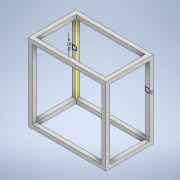
# Autodesk Inventor part: Battery housing
Saved by Autodesk Inventor 2020 (Build 240168000, 168)
## iProperties
Created: 2020-10-20
Part Number: Battery housing
Material: Generic
Document SubType Name: Modeling
Designer: jtri402
Density: 1 g/cm^3
Appearance: Default
Author: jtri402
Autodesk Inventor part; units mm, degrees
ref_plane "YZ Plane" through (0, 0, 0) normal (1, 0, 0) x (0, 1, 0)
ref_plane "XZ Plane" through (0, 0, 0) normal (0, 1, 0) x (-1, 0, 0)
ref_plane "XY Plane" through (0, 0, 0) normal (0, 0, 1) x (1, 0, 0)
sketch "Sketch1" plane through (0, 0, 0) normal (0, 0, 1) x (1, 0, 0)
  line L0 (0, 0) -> (175, 0)
  line L1 (175, 0) -> (175, 175)
  line L2 (175, 175) -> (0, 175)
  line L3 (0, 175) -> (0, 0)
  dimension "d0" = 175
  dimension "d1" = 175
  constraints: 8 end point, 2 parallel, 1 horizontal, 1 perpendicular
  measures "d0" distance of L2.end L0.start
  measures "d1" distance of L0.start L0.end
extrude "Extrusion1" add sketch "Sketch1" along normal blind 100
sketch "Sketch2" plane through (0, 175, 0) normal (0, 1, 0) x (1, 0, 0)
  line L0 (0, 0) -> (175, 0) projected
  line L1 (0, -100) -> (175, -100) projected
  line L2 (0, 0) -> (175, 0)
  line L3 (175, 0) -> (175, -100)
  line L4 (175, -100) -> (0, -100)
  line L5 (0, -100) -> (0, 0)
  line L6 (10, -10) -> (165, -10)
  line L7 (165, -10) -> (165, -90)
  line L8 (165, -90) -> (10, -90)
  line L9 (10, -90) -> (10, -10)
  dimension "d4" = 10
  dimension "d5" = 10
  dimension "d6" = 10
  dimension "d7" = 10
  constraints: 16 end point, 4 parallel, 2 horizontal, 2 perpendicular
  measures "d4" distance between parallel lines of L0 L6
  measures "d5" distance between parallel lines of L5 L9
  measures "d6" distance between parallel lines of L1 L8
  measures "d7" distance between parallel lines of L3 L7
extrude "Extrusion2" add sketch "Sketch2" along normal blind 10
sketch "Sketch3" plane through (10, 175, 10) normal (0, 1, 0) x (1, 0, 0)
  line L0 (0, -80) -> (0, 0) projected
  line L1 (0, -80) -> (155, -80) projected
  line L2 (0, 0) -> (155, 0)
  line L3 (155, 0) -> (155, -80)
  line L4 (155, -80) -> (0, -80)
  line L5 (0, -80) -> (0, 0)
  point P0 (-10, 10)
  constraints: 8 end point, 2 parallel, 1 horizontal, 1 perpendicular
extrude "Extrusion3" cut sketch "Sketch3" against normal blind 9000
sketch "Sketch4" plane through (0, 0, 100) normal (0, 0, 1) x (1, 0, 0)
  line L0 (175, 0) -> (175, 185) projected
  line L1 (175, 185) -> (195, 185)
  line L2 (195, 185) -> (195, 0)
  line L3 (195, 0) -> (175, 0)
  line L4 (175, 0) -> (175, 185)
  point P0 (0, 0)
  dimension "d12" = 20
  constraints: 8 end point, 2 parallel, 1 horizontal, 1 perpendicular
  measures "d12" distance of L2.end L3.end
extrude "Extrusion4" add sketch "Sketch4" against normal blind 100
sketch "Sketch5" plane through (0, 0, 100) normal (0, 0, 1) x (1, 0, 0)
  line L0 (10, 175) -> (185, 175)
  line L1 (185, 175) -> (185, 10)
  line L2 (185, 10) -> (10, 10)
  line L3 (10, 10) -> (10, 175)
  line L4 (0, 185) -> (195, 185) projected
  line L5 (0, 0) -> (0, 185) projected
  line L6 (0, 0) -> (195, 0) projected
  line L7 (195, 0) -> (195, 185) projected
  dimension "d15" = 10
  dimension "d16" = 10
  dimension "d17" = 10
  dimension "d18" = 10
  constraints: 8 end point, 2 parallel, 1 horizontal, 1 perpendicular
  measures "d15" distance between parallel lines of L4 L0
  measures "d16" distance between parallel lines of L5 L3
  measures "d17" distance between parallel lines of L6 L2
  measures "d18" distance between parallel lines of L7 L1
extrude "Extrusion5" cut sketch "Sketch5" against normal blind 100 contours L0 L1 L2 L3
sketch "Sketch6" plane through (195, 0, 100) normal (1, 0, 0) x (0, 0, -1)
  point P0 (100, 0)
sketch "Sketch7" plane through (0, 185, 0) normal (0, 1, 0) x (1, 0, 0)
  line L0 (0, -100) -> (195, -100) projected
  line L1 (0, 0) -> (195, 0)
  line L2 (195, 0) -> (195, -100)
  line L3 (195, -100) -> (0, -100)
  line L4 (0, -100) -> (0, 0)
  constraints: 8 end point, 2 parallel, 1 horizontal, 1 perpendicular
extrude "Extrusion6" add sketch "Sketch7" along normal blind 10
sketch "Sketch8" plane through (0, 195, 0) normal (0, 1, 0) x (1, 0, 0)
  line L0 (10, -10) -> (10, 0) projected
  line L1 (10, -10) -> (185, -10)
  line L2 (185, -10) -> (185, -90)
  line L3 (185, -90) -> (10, -90)
  line L4 (10, -90) -> (10, -10)
  line L5 (0, -100) -> (195, -100) projected
  line L6 (195, -100) -> (195, 0) projected
  point P0 (0, 0)
  dimension "d23" = 10
  dimension "d24" = 10
  constraints: 8 end point, 2 parallel, 1 horizontal, 1 perpendicular
  measures "d23" distance between parallel lines of L5 L3
  measures "d24" distance between parallel lines of L6 L2
extrude "Extrusion7" cut sketch "Sketch8" against normal blind 900
sketch "Sketch9" plane through (195, 0, 100) normal (1, 0, 0) x (0, 0, -1)
  line L0 (10, 185) -> (90, 185)
  line L1 (90, 185) -> (90, 10)
  line L2 (90, 10) -> (10, 10)
  line L3 (10, 10) -> (10, 185)
  line L4 (0, 195) -> (100, 195) projected
  line L5 (0, 0) -> (0, 195) projected
  line L6 (0, 0) -> (100, 0) projected
  line L7 (100, 0) -> (100, 195) projected
  dimension "d27" = 10
  dimension "d28" = 10
  dimension "d29" = 10
  dimension "d30" = 10
  constraints: 8 end point, 2 parallel, 1 horizontal, 1 perpendicular
  measures "d27" distance between parallel lines of L4 L0
  measures "d28" distance between parallel lines of L5 L3
  measures "d29" distance between parallel lines of L6 L2
  measures "d30" distance between parallel lines of L7 L1
extrude "Extrusion8" cut sketch "Sketch9" against normal blind 900 contours L0 L1 L2 L3
sketch "Sketch10" plane through (0, 0, 100) normal (0, 0, 1) x (1, 0, 0)
  line L0 (185, 175) -> (10, 175) projected
  line L1 (185, 195) -> (185, 185) projected
  line L2 (10, 175) -> (185, 175)
  line L3 (185, 175) -> (185, 185)
  line L4 (185, 185) -> (10, 185)
  line L5 (10, 185) -> (10, 175)
  point P0 (0, 0)
  constraints: 8 end point, 2 parallel, 1 horizontal, 1 perpendicular
extrude "Extrusion9" cut sketch "Sketch10" against normal blind 900
sketch "Sketch11" plane through (0, 0, 100) normal (0, 0, 1) x (1, 0, 0)
  line L0 (0, 0) -> (0, 195) projected
  line L1 (0, 0) -> (195, 0) projected
  line L2 (0, 195) -> (195, 195)
  line L3 (195, 195) -> (195, 0)
  line L4 (195, 0) -> (0, 0)
  line L5 (0, 0) -> (0, 195)
  line L6 (10, 185) -> (10, 10) projected
  line L7 (185, 10) -> (10, 10) projected
  line L8 (10, 185) -> (185, 185)
  line L9 (185, 185) -> (185, 10)
  line L10 (185, 10) -> (10, 10)
  line L11 (10, 10) -> (10, 185)
  constraints: 16 end point, 4 parallel, 2 horizontal, 2 perpendicular
extrude "Extrusion10" add sketch "Sketch11" along normal blind 20
sketch "Sketch12" plane through (0, 195, 0) normal (0, 1, 0) x (1, 0, 0)
  line L0 (10, -90) -> (0, -90) projected
  line L1 (185, -120) -> (185, -90) projected
  line L2 (10, -90) -> (185, -90)
  line L3 (185, -90) -> (185, -110)
  line L4 (185, -110) -> (10, -110)
  line L5 (10, -110) -> (10, -90)
  line L6 (195, -120) -> (0, -120) projected
  point P0 (0, 0)
  dimension "d37" = 10
  constraints: 8 end point, 2 parallel, 1 horizontal, 1 perpendicular, 1 point on line
  measures "d37" distance between parallel lines of L6 L4
extrude "Extrusion11" cut sketch "Sketch12" against normal blind 900
sketch "Sketch13" plane through (195, 0, 0) normal (1, 0, 0) x (0, 0, -1)
  line L0 (-90, 185) -> (-10, 185) projected
  line L1 (-120, 10) -> (-110, 10) projected
  line L2 (-90, 185) -> (-110, 185)
  line L3 (-110, 185) -> (-110, 10)
  line L4 (-110, 10) -> (-90, 10)
  line L5 (-90, 10) -> (-90, 185)
  point P0 (0, 0)
  constraints: 8 end point, 2 parallel, 1 horizontal, 1 perpendicular
extrude "Extrusion12" cut sketch "Sketch13" against normal blind 900
sketch "Sketch15" plane through (0, 10, 10) normal (0, 0, 1) x (1, 0, 0)
  line L0 (10, 175) -> (10, 0) projected
  line L1 (0, 115) -> (10, 115)
  line L2 (10, 115) -> (10, 105)
  line L3 (10, 105) -> (0, 105)
  line L4 (0, 105) -> (0, 115)
  point P0 (10, 115)
  point P1 (10, 115)
  dimension "d45" = 10
  constraints: 8 end point, 2 parallel, 1 horizontal, 1 perpendicular, 1 point on line
  measures "d45" distance of L3.end L1.start
sketch "Sketch16" plane through (185, 10, 10) normal (0, 0, 1) x (1, 0, 0)
  line L0 (0, 115) -> (10, 115) projected
  line L1 (0, 115) -> (10, 115)
  line L2 (10, 115) -> (10, 105)
  line L3 (10, 105) -> (0, 105)
  line L4 (0, 105) -> (0, 115)
  point P0 (-185, -10)
  point P1 (10, 115)
  dimension "d46" = 10
  constraints: 8 end point, 2 parallel, 1 horizontal, 1 perpendicular
  measures "d46" distance of L1.end L2.end
body "Solid1"
